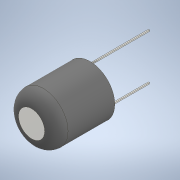
# Autodesk Inventor part: bulb
Saved by Autodesk Inventor 2021 (Build 250183000, 183)
## iProperties
Created: 2021-07-30
Part Number: bulb
Material: Glass
Document SubType Name: Modeling
Designer: user
Density: 2.18 g/cm^3
Appearance: Clear
Author: user
Autodesk Inventor part; units mm, degrees
ref_plane "YZ Plane" through (0, 0, 0) normal (1, 0, 0) x (0, 1, 0)
ref_plane "XZ Plane" through (0, 0, 0) normal (0, 1, 0) x (-1, 0, 0)
ref_plane "XY Plane" through (0, 0, 0) normal (0, 0, 1) x (1, 0, 0)
sketch "Sketch1" plane through (0, 0, 0) normal (0, 0, 1) x (1, 0, 0)
  circle A0 centre (0, 0) radius 4.2426
  constraints: 1 centre point, 1 coincident
extrude "Extrusion1" add sketch "Sketch1" along normal blind 10
fillet "Fillet1" radius 2 1 edges at (-4.2426, 0, 10)
sketch "Sketch2" plane through (0, 0, 0) normal (0, 0, -1) x (-1, 0, 0)
  line L0 (0, -4) -> (-0.2, -4)
  line L1 (-0.2, -4) -> (-0.2, -3.8)
  line L2 (-0.2, -3.8) -> (0, -3.8)
  line L3 (0, -3.8) -> (0, -4)
  line L4 (0, 4) -> (-0.2, 4)
  line L5 (-0.2, 4) -> (-0.2, 3.8)
  line L6 (-0.2, 3.8) -> (0, 3.8)
  line L7 (0, 3.8) -> (0, 4)
  point P0 (0, 0)
  dimension "d3" = 0.2
  dimension "d4" = 0.2
  dimension "d5" = 0.2
  dimension "d6" = 0.2
  constraints: 16 end point, 4 parallel, 2 horizontal, 2 perpendicular
  measures "d3" distance of L1.end L2.end
  measures "d4" distance of L0.end L1.end
  measures "d5" distance of L6.end L5.end
  measures "d6" distance of L5.end L4.end
extrude "Extrusion2" add sketch "Sketch2" along normal blind 10 contours L0 L1 L2 L3
sketch "Sketch3" plane through (0, 0, 0) normal (0, 0, -1) x (-1, 0, 0)
  point P0 (0, 0)
sketch "Sketch4" plane through (0, 0, 0) normal (0, 0, -1) x (-1, 0, 0)
  line L0 (0, 4) -> (-0.2, 4)
  line L1 (-0.2, 4) -> (-0.2, 3.8)
  line L2 (-0.2, 3.8) -> (0, 3.8)
  line L3 (0, 3.8) -> (0, 4)
  point P0 (0, 0)
  dimension "d9" = 0.2
  dimension "d10" = 0.2
  constraints: 8 end point, 2 parallel, 1 horizontal, 1 perpendicular
  measures "d9" distance of L2.end L1.end
  measures "d10" distance of L1.end L0.end
extrude "Extrusion3" add sketch "Sketch4" along normal blind 10
body "Solid1"
